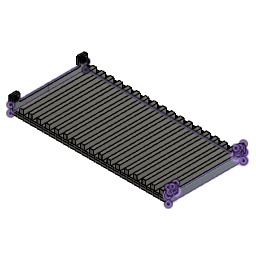
SSDTray v8 (Autodesk Fusion 360 archive; units mm, degrees)
design "SSDTray-Top"
Autodesk Fusion 360 part; units mm, degrees
sketch "PrimarySSD" plane through (0, 0, 0) normal (0, 1, 0) x (1, 0, 0)
  line L0 (0, 0) -> (7, 0)
  circle A0 centre (4, -14) radius 1.55
  circle A1 centre (4, -90.6) radius 1.55
  line L1 (0, 0) -> (-2.5, 0)
  line L2 (-2.5, 0) -> (-2.5, -100.45)
  line L3 (0, -100.45) -> (0, 0)
  line L4 (7, 0) -> (9.5, 0)
  line L5 (9.5, 0) -> (9.5, -100.45)
  line L6 (7, -100.45) -> (7, 0)
  line L7 (-2.5, -100.45) -> (9.5, -100.45)
  line L8 (-2.5, -100.45) -> (9.5, -100.45)
  line L9 (9.5, -100.45) -> (9.5, -102.95)
  line L10 (9.5, -102.95) -> (-2.5, -102.95)
  line L11 (-2.5, -102.95) -> (-2.5, -100.45)
  dimension "d1" = 7
  dimension "d3" = 3.1
  dimension "d5" = 14
  dimension "d6" = 3.1
  dimension "d8" = 90.6
  dimension "d10" = 100.45
  dimension "d12" = 100.45
  dimension "d17" = 2.5
  dimension "d18" = 2.5
  dimension "d19" = 12
  dimension "d20" = 3
  dimension "d21" = 3
  dimension "d44" = 9.85
  dimension "d92" = 12
  dimension "d93" = 2.5
  constraint horizontal L0
  constraint coincident L0.start L1.start
  constraint horizontal L1
  constraint vertical L2
  constraint vertical L3
  constraint horizontal L4
  constraint vertical L5
  constraint vertical L6
  constraint perpendicular L5 L7
  constraint horizontal L8
  constraint vertical L9
  constraint horizontal L10
  constraint vertical L11
  measures "d1" distance of L0.start L0.end
  measures "d3" diameter of A0
  measures "d5" distance of L0 A0.centre
  measures "d6" diameter of A1
  measures "d8" distance of L0 A1.centre
  measures "d10" distance of L0.start L3.start
  measures "d12" distance of L0.end L6.start
  measures "d17" distance of L2 L3
  measures "d18" distance of L5 L6
  measures "d19" distance of L2 L5
  measures "d20" distance of A1.centre L6
  measures "d21" distance of A0.centre L6
  measures "d44" distance of A1.centre L7
  measures "d92" distance of L2.end L5.end
  measures "d93" distance of L2.end L10.end
extrude "Extrude1" add sketch "PrimarySSD" along normal blind 10 contours L1 L2 L3 L7 L8 | L4 L5 L6 L7 L8 makes body 1 at (0, 3.3333, 66.9667) makes body 2 at (9.5, 3.3333, 33.4833)
extrude "Extrude6" add sketch "PrimarySSD" along normal blind 3 contours L0 L3 L6 L7 L8 bodies 1 2
ref_plane "WorkPlane2" through (3.5, 72.85, 50.225) normal (0, 1, 0) x (1, 0, 0)
sketch "TopSSD" plane through (0, 72.85, 0) normal (0, 1, 0) x (1, 0, 0)
  line L0 (-2.5, 0) -> (-2.5, -100.45)
  line L1 (0, -100.45) -> (0, 0)
  line L2 (7, -100.45) -> (7, 0)
  line L3 (9.5, 0) -> (9.5, -100.45)
  line L4 (-2.5, -100.45) -> (9.5, -100.45)
  line L5 (0, 0) -> (7, 0)
  line L6 (7, 0) -> (9.5, 0)
  line L7 (0, 0) -> (-2.5, 0)
  circle A0 centre (4, -14) radius 1.55
  circle A1 centre (4, -90.6) radius 1.55
  line L8 (9.5, -102.95) -> (-2.5, -102.95)
  line L9 (9.5, -100.45) -> (9.5, -102.95)
  line L10 (-2.5, -102.95) -> (-2.5, -100.45)
  point P0 (4, -14)
  point P1 (4, -90.6)
  point P2 (9.5, 0)
  point P3 (-2.5, 0)
  point P4 (9.5, -100.45)
extrude "Extrude12" add sketch "PrimarySSD" along normal blind 10 contours L7 L8 L9 L10 L11 bodies 1
pattern_linear "R-Pattern1" count 18 spacing 12 along (1, 0, 0) of bodies 1 makes body 3 at (15.6281, 0, 4.1514) makes body 4 at (27.6281, 0, 4.1514) makes body 5 at (39.6281, 0, 4.1514) makes body 6 at (51.6281, 0, 4.1514) makes body 7 at (63.6281, 0, 4.1514) makes body 8 at (75.6281, 0, 4.1514) makes body 9 at (87.6281, 0, 4.1514) makes body 10 at (99.6281, 0, 4.1514) makes body 11 at (111.6281, 0, 4.1514) makes body 12 at (123.6281, 0, 4.1514) makes body 13 at (135.6281, 0, 4.1514) makes body 14 at (147.6281, 0, 4.1514) makes body 15 at (159.6281, 0, 4.1514) makes body 16 at (171.6281, 0, 4.1514) makes body 17 at (183.6281, 0, 4.1514) makes body 18 at (195.6281, 0, 4.1514) makes body 19 at (207.6281, 0, 4.1514)
combine "Combine6" operation add target body 1 tool bodies 3 13 17 16 18 19 10 11 14 5 6 15 9 8 7 4 12
ref_plane "WorkPlane5" through (-2.5, 5, 51.475) normal (-1, 0, 0) x (0, 0, 1)
sketch "Left Mount" plane through (-2.5, 0, 0) normal (-1, 0, 0) x (0, 0, 1)
  line L0 (0, 0) -> (102.95, 0)
  line L1 (102.95, 0) -> (102.95, 10)
  line L2 (102.95, 10) -> (0, 10)
  line L3 (0, 10) -> (0, 0)
  line L4 (0, 10) -> (10, 10)
  line L5 (10, 10) -> (10, 20)
  line L6 (10, 20) -> (0, 20)
  line L7 (0, 20) -> (0, 10)
  line L8 (51.475, 0) -> (51.475, 10)
  line L9 (102.95, 20) -> (102.95, 10)
  line L10 (92.95, 20) -> (102.95, 20)
  line L11 (102.95, 10) -> (92.95, 10)
  line L12 (92.95, 10) -> (92.95, 20)
  circle A0 centre (5, 15) radius 1.625
  circle A1 centre (97.95, 15) radius 1.625
  line L13 (7.75, 16.5877) -> (5, 18.1754)
  line L14 (5, 18.1754) -> (2.25, 16.5877)
  line L15 (2.25, 16.5877) -> (2.25, 13.4123)
  line L16 (2.25, 13.4123) -> (5, 11.8246)
  line L17 (5, 11.8246) -> (7.75, 13.4123)
  line L18 (7.75, 13.4123) -> (7.75, 16.5877)
  line L19 (95.2, 16.5877) -> (97.95, 18.1754)
  line L20 (97.95, 18.1754) -> (100.7, 16.5877)
  line L21 (100.7, 16.5877) -> (100.7, 13.4123)
  line L22 (100.7, 13.4123) -> (97.95, 11.8246)
  line L23 (97.95, 11.8246) -> (95.2, 13.4123)
  line L24 (95.2, 13.4123) -> (95.2, 16.5877)
  point P0 (5, 15)
  dimension "d103" = 10
  dimension "d104" = 10
  dimension "d105" = 3.25
  dimension "d106" = 5
  dimension "d107" = 5
  dimension "d108" = 2.75
  constraint horizontal L4
  constraint vertical L5
  constraint horizontal L6
  constraint vertical L7
  constraint coincident L2.end L3.start
  constraint midpoint L0 L8.start
  constraint midpoint L2 L8.end
  constraint symmetric L2.end L8 L1.end
  constraint symmetric L4.end L8 L11.end
  constraint symmetric L5.end L8 L10.start
  constraint symmetric L6.end L8 L9.start
  constraint symmetric L8 A0 A1
  constraint coincident P0 A0.centre
  constraint vertical L15
  constraint symmetric L8 L13.start L19.start
  constraint symmetric L8 L13.end L19.end
  constraint symmetric L8 L14.end L20.end
  constraint symmetric L8 L15.end L21.end
  constraint symmetric L8 L16.end L22.end
  constraint symmetric L8 L17.end L23.end
  measures "d103" distance of L2.end L4.end
  measures "d104" distance of L2.end L6.end
  measures "d105" diameter of A0
  measures "d106" distance of L7 P0
  measures "d107" distance of L6 P0
  measures "d108" distance of P0 L18
extrude "Extrude15" add sketch "Left Mount" against normal blind 2.5 contours L2 L4 L5 L6 L7 bodies 1
extrude "Extrude16" add sketch "Left Mount" against normal blind 2.5 contours L2 L9 L10 L11 L12 bodies 1
extrude "Extrude17" add sketch "Left Mount" along normal blind 2.5 contours L2 L9 L10 L11 L12 | L19 L20 L21 L22 L23 L24 bodies 1
extrude "Extrude18" add sketch "Left Mount" along normal blind 2.5 contours L2 L4 L5 L6 L7 | L13 L14 L15 L16 L17 L18 bodies 1
ref_plane "WorkPlane6" through (213.5, 5, 51.475) normal (1, 0, 0) x (0, 0, -1)
sketch "Right Mount" plane through (213.5, 0, 0) normal (1, 0, 0) x (0, 0, -1)
  line L0 (-102.95, 0) -> (-102.95, 10)
  line L1 (0, 0) -> (-102.95, 0)
  line L2 (-102.95, 10) -> (0, 10)
  line L3 (0, 10) -> (0, 0)
  line L4 (0, 20) -> (0, 10)
  line L5 (-2.25, 16.5877) -> (-2.25, 13.4123)
  line L6 (-2.25, 13.4123) -> (-5, 11.8246)
  line L7 (-5, 11.8246) -> (-7.75, 13.4123)
  line L8 (-7.75, 13.4123) -> (-7.75, 16.5877)
  line L9 (-7.75, 16.5877) -> (-5, 18.1754)
  line L10 (-5, 18.1754) -> (-2.25, 16.5877)
  circle A0 centre (-5, 15) radius 1.625
  line L11 (-10, 20) -> (0, 20)
  line L12 (-10, 10) -> (-10, 20)
  line L13 (-92.95, 10) -> (-92.95, 20)
  line L14 (-92.95, 20) -> (-102.95, 20)
  line L15 (-102.95, 20) -> (-102.95, 10)
  line L16 (-100.7, 16.5877) -> (-100.7, 13.4123)
  line L17 (-100.7, 13.4123) -> (-97.95, 11.8246)
  line L18 (-97.95, 11.8246) -> (-95.2, 13.4123)
  line L19 (-95.2, 13.4123) -> (-95.2, 16.5877)
  line L20 (-95.2, 16.5877) -> (-97.95, 18.1754)
  line L21 (-97.95, 18.1754) -> (-100.7, 16.5877)
  circle A1 centre (-97.95, 15) radius 1.625
  point P0 (-5, 15)
  point P1 (-97.95, 15)
extrude "Extrude19" add sketch "Right Mount" against normal blind 2.5 contours L2 L13 L14 L15 bodies 1
extrude "Extrude20" add sketch "Right Mount" along normal blind 2.5 contours L2 L13 L14 L15 | L16 L17 L18 L19 L20 L21 bodies 1
extrude "Extrude21" add sketch "Right Mount" against normal blind 2.5 contours L2 L4 L11 L12 bodies 1
extrude "Extrude22" add sketch "Right Mount" along normal blind 2.5 contours L2 L4 L11 L12 | L5 L6 L7 L8 L9 L10 bodies 1
sketch "Sketch13" plane through (0, 10, 0) normal (0, 1, 0) x (-1, 0, 0)
  line L0 (-211, 102.95) -> (-211, 100.45)
  line L1 (-211, 100.45) -> (-204, 100.45)
  line L2 (-204, 100.45) -> (-204, 0)
  line L3 (-204, 0) -> (-199, 0)
  line L4 (-199, 0) -> (-199, 100.45)
  line L5 (-199, 100.45) -> (-192, 100.45)
  line L6 (-192, 100.45) -> (-192, 0)
  line L7 (-192, 0) -> (-187, 0)
  line L8 (-187, 0) -> (-187, 100.45)
  line L9 (-187, 100.45) -> (-180, 100.45)
  line L10 (-180, 100.45) -> (-180, 0)
  line L11 (-180, 0) -> (-175, 0)
  line L12 (-175, 0) -> (-175, 100.45)
  line L13 (-175, 100.45) -> (-168, 100.45)
  line L14 (-168, 100.45) -> (-168, 0)
  line L15 (-168, 0) -> (-163, 0)
  line L16 (-163, 0) -> (-163, 100.45)
  line L17 (-163, 100.45) -> (-156, 100.45)
  line L18 (-156, 100.45) -> (-156, 0)
  line L19 (-156, 0) -> (-151, 0)
  line L20 (-151, 0) -> (-151, 100.45)
  line L21 (-151, 100.45) -> (-144, 100.45)
  line L22 (-144, 100.45) -> (-144, 0)
  line L23 (-144, 0) -> (-139, 0)
  line L24 (-139, 0) -> (-139, 100.45)
  line L25 (-139, 100.45) -> (-132, 100.45)
  line L26 (-132, 100.45) -> (-132, 0)
  line L27 (-132, 0) -> (-127, 0)
  line L28 (-127, 0) -> (-127, 100.45)
  line L29 (-127, 100.45) -> (-120, 100.45)
  line L30 (-120, 100.45) -> (-120, 0)
  line L31 (-120, 0) -> (-115, 0)
  line L32 (-115, 0) -> (-115, 100.45)
  line L33 (-115, 100.45) -> (-108, 100.45)
  line L34 (-108, 100.45) -> (-108, 0)
  line L35 (-108, 0) -> (-103, 0)
  line L36 (-103, 0) -> (-103, 100.45)
  line L37 (-103, 100.45) -> (-96, 100.45)
  line L38 (-96, 100.45) -> (-96, 0)
  line L39 (-96, 0) -> (-91, 0)
  line L40 (-91, 0) -> (-91, 100.45)
  line L41 (-91, 100.45) -> (-84, 100.45)
  line L42 (-84, 100.45) -> (-84, 0)
  line L43 (-84, 0) -> (-79, 0)
  line L44 (-79, 0) -> (-79, 100.45)
  line L45 (-79, 100.45) -> (-72, 100.45)
  line L46 (-72, 100.45) -> (-72, 0)
  line L47 (-72, 0) -> (-67, 0)
  line L48 (-67, 0) -> (-67, 100.45)
  line L49 (-67, 100.45) -> (-60, 100.45)
  line L50 (-60, 100.45) -> (-60, 0)
  line L51 (-60, 0) -> (-55, 0)
  line L52 (-55, 0) -> (-55, 100.45)
  line L53 (-55, 100.45) -> (-48, 100.45)
  line L54 (-48, 100.45) -> (-48, 0)
  line L55 (-48, 0) -> (-43, 0)
  line L56 (-43, 0) -> (-43, 100.45)
  line L57 (-43, 100.45) -> (-36, 100.45)
  line L58 (-36, 100.45) -> (-36, 0)
  line L59 (-36, 0) -> (-31, 0)
  line L60 (-31, 0) -> (-31, 100.45)
  line L61 (-31, 100.45) -> (-24, 100.45)
  line L62 (-24, 100.45) -> (-24, 0)
  line L63 (-24, 0) -> (-19, 0)
  line L64 (-19, 0) -> (-19, 100.45)
  line L65 (-19, 100.45) -> (-12, 100.45)
  line L66 (-12, 100.45) -> (-12, 0)
  line L67 (-12, 0) -> (-7, 0)
  line L68 (-7, 0) -> (-7, 100.45)
  line L69 (-7, 100.45) -> (0, 100.45)
  line L70 (0, 100.45) -> (0, 102.95)
  line L71 (0, 102.95) -> (-211, 102.95)
  line L72 (2.5, 102.95) -> (-15.75, 102.95)
  line L73 (-7, 100.45) -> (0, 100.45)
  line L74 (-19, 100.45) -> (-12, 100.45)
  line L75 (-211, 102.95) -> (0, 102.95)
  line L76 (-31, 100.45) -> (-24, 100.45)
  line L77 (-43, 100.45) -> (-36, 100.45)
  line L78 (0, 102.95) -> (-211, 102.95)
  line L79 (-211, 102.95) -> (-211, 100.45)
  line L80 (-211, 100.45) -> (0, 100.45)
  line L81 (0, 100.45) -> (0, 102.95)
  line L82 (-211, 102.95) -> (-211, 100.45)
  line L83 (-211, 100.45) -> (-204, 100.45)
  line L84 (-204, 100.45) -> (-204, 0)
  line L85 (-204, 0) -> (-199, 0)
  line L86 (-199, 0) -> (-199, 100.45)
  line L87 (-199, 100.45) -> (-192, 100.45)
  line L88 (-192, 100.45) -> (-192, 0)
  line L89 (-192, 0) -> (-187, 0)
  line L90 (-187, 0) -> (-187, 100.45)
  line L91 (-187, 100.45) -> (-180, 100.45)
  line L92 (-180, 100.45) -> (-180, 0)
  line L93 (-180, 0) -> (-175, 0)
  line L94 (-175, 0) -> (-175, 100.45)
  line L95 (-175, 100.45) -> (-168, 100.45)
  line L96 (-168, 100.45) -> (-168, 0)
  line L97 (-168, 0) -> (-163, 0)
  line L98 (-163, 0) -> (-163, 100.45)
  line L99 (-163, 100.45) -> (-156, 100.45)
  line L100 (-156, 100.45) -> (-156, 0)
  line L101 (-156, 0) -> (-151, 0)
  line L102 (-151, 0) -> (-151, 100.45)
  line L103 (-151, 100.45) -> (-144, 100.45)
  line L104 (-144, 100.45) -> (-144, 0)
  line L105 (-144, 0) -> (-139, 0)
  line L106 (-139, 0) -> (-139, 100.45)
  line L107 (-139, 100.45) -> (-132, 100.45)
  line L108 (-132, 100.45) -> (-132, 0)
  line L109 (-132, 0) -> (-127, 0)
  line L110 (-127, 0) -> (-127, 100.45)
  line L111 (-127, 100.45) -> (-120, 100.45)
  line L112 (-120, 100.45) -> (-120, 0)
  line L113 (-120, 0) -> (-115, 0)
  line L114 (-115, 0) -> (-115, 100.45)
  line L115 (-115, 100.45) -> (-108, 100.45)
  line L116 (-108, 100.45) -> (-108, 0)
  line L117 (-108, 0) -> (-103, 0)
  line L118 (-103, 0) -> (-103, 100.45)
  line L119 (-103, 100.45) -> (-96, 100.45)
  line L120 (-96, 100.45) -> (-96, 0)
  line L121 (-96, 0) -> (-91, 0)
  line L122 (-91, 0) -> (-91, 100.45)
  line L123 (-91, 100.45) -> (-84, 100.45)
  line L124 (-84, 100.45) -> (-84, 0)
  line L125 (-84, 0) -> (-79, 0)
  line L126 (-79, 0) -> (-79, 100.45)
  line L127 (-79, 100.45) -> (-72, 100.45)
  line L128 (-72, 100.45) -> (-72, 0)
  line L129 (-72, 0) -> (-67, 0)
  line L130 (-67, 0) -> (-67, 100.45)
  line L131 (-67, 100.45) -> (-60, 100.45)
  line L132 (-60, 100.45) -> (-60, 0)
  line L133 (-60, 0) -> (-55, 0)
  line L134 (-55, 0) -> (-55, 100.45)
  line L135 (-55, 100.45) -> (-48, 100.45)
  line L136 (-48, 100.45) -> (-48, 0)
  line L137 (-48, 0) -> (-43, 0)
  line L138 (-43, 0) -> (-43, 100.45)
  line L139 (-43, 100.45) -> (-36, 100.45)
  line L140 (-36, 100.45) -> (-36, 0)
  line L141 (-36, 0) -> (-31, 0)
  line L142 (-31, 0) -> (-31, 100.45)
  line L143 (-31, 100.45) -> (-24, 100.45)
  line L144 (-24, 100.45) -> (-24, 0)
  line L145 (-24, 0) -> (-19, 0)
  line L146 (-19, 0) -> (-19, 100.45)
  line L147 (-19, 100.45) -> (-12, 100.45)
  line L148 (-12, 100.45) -> (-12, 0)
  line L149 (-12, 0) -> (-7, 0)
  line L150 (-7, 0) -> (-7, 100.45)
  line L151 (-7, 100.45) -> (0, 100.45)
  line L152 (0, 100.45) -> (0, 102.95)
  line L153 (0, 102.95) -> (-211, 102.95)
  dimension "d187" = 211
  dimension "d188" = 2.5
  constraint horizontal L78
  constraint vertical L79
  constraint horizontal L80
  constraint vertical L81
  constraint coincident L70.end L71.start
  measures "d187" distance of L70.end L0.start
  measures "d188" distance of L70.end L69.end
extrude "Extrude35" cut sketch "Sketch13" against normal blind 6.5 contours L0 L1 L5 L9 L13 L17 L21 L25 L29 L33 L37 L41 L45 L49 L53 L57 L61 L65 L69 L70 L71 L72 L73 L74 L75 L76 L77 L78 L79 L80 L81 L82 L83 L87 L91 L95 L99 L103 L107 L111 L115 L119 L123 L127 L131 L135 L139 L143 L147 L151 L152 L153 bodies 1
sketch "Sketch14" plane through (0, 0, 0) normal (0, 1, 0) x (1, 0, 0)
  line L0 (-2.5, 0) -> (213.5, 0)
  line L1 (-2.5, 0) -> (213.5, 0)
  line L2 (213.5, 0) -> (213.5, 1.6)
  line L3 (213.5, 1.6) -> (-2.5, 1.6)
  line L4 (-2.5, 1.6) -> (-2.5, 0)
  line L5 (-2.5, 0) -> (213.5, 0)
  line L6 (213.5, 0) -> (213.5, 2.5)
  line L7 (213.5, 2.5) -> (-2.5, 2.5)
  line L8 (-2.5, 2.5) -> (-2.5, 0)
  dimension "d191" = 216
  dimension "d192" = 1.6
  dimension "d193" = 2.5
  constraint horizontal L1
  constraint vertical L2
  constraint horizontal L3
  constraint vertical L4
  constraint coincident L0.start L1.start
  constraint horizontal L5
  constraint vertical L6
  constraint horizontal L7
  constraint vertical L8
  measures "d191" distance of L0.start L0.end
  measures "d192" distance of L0.start L3.end
  measures "d193" distance of L0.start L7.end
extrude "Extrude36" add sketch "Sketch14" along normal blind 3 bodies 1
extrude "Extrude37" add sketch "Sketch14" along normal blind 5 contours L3 L6 L7 L8 bodies 1
named bodies: "BottomTray"

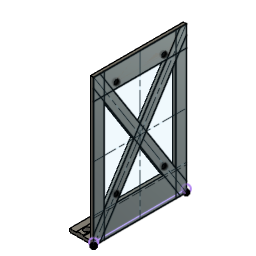
design "2U Ears"
Autodesk Fusion 360 part; units mm, degrees
sketch "Sketch1" plane through (0, 0, 0) normal (0, 1, 0) x (1, 0, 0)
  line L0 (0, 0) -> (-20, 0)
  line L1 (-20, 0) -> (-20, -44.45)
  line L2 (-20, -44.45) -> (0, -44.45)
  line L3 (0, -44.45) -> (0, 0)
  line L4 (-10, 0) -> (-10, -44.45)
  circle A0 centre (-10, -6.35) radius 3.05
  circle A1 centre (-10, -22.225) radius 3.05
  circle A2 centre (-10, -38.1) radius 3.05
  line L5 (-6.9, -44.45) -> (-13.1, -44.45)
  line L6 (-13.1, -44.45) -> (-13.1, 0)
  line L7 (-13.1, 0) -> (-6.9, 0)
  line L8 (-6.9, 0) -> (-6.9, -44.45)
  line L9 (-6.9, -44.45) -> (-13.1, 0) construction
  line L10 (-13.1, -44.45) -> (-6.9, 0) construction
  line L11 (0, 0) -> (3, 0)
  line L12 (3, 0) -> (3, -44.45)
  line L13 (3, -44.45) -> (0, -44.45)
  line L14 (0, -44.45) -> (0, 0)
  point P0 (-10, -22.225)
  dimension "d1" = 20
  dimension "d2" = 44.45
  dimension "d3" = 6.1
  dimension "d4" = 6.35
  dimension "d5" = 6.1
  dimension "d6" = 15.875
  dimension "d7" = 6.1
  dimension "d8" = 15.875
  dimension "d9" = 6.35
  dimension "d10" = 6.2
  dimension "d11" = 44.45
  dimension "d12" = 3
  dimension "d13" = 44.45
  constraint horizontal L0
  constraint vertical L1
  constraint horizontal L2
  constraint vertical L3
  constraint coincident L0.start L3.end
  constraint midpoint L0 L4.start
  constraint midpoint L2 L4.end
  constraint coincident L4 A0.centre
  constraint coincident L4 P0
  constraint coincident L4 A2.centre
  constraint horizontal L5
  constraint perpendicular L5 L6
  constraint parallel L5 L7
  constraint parallel L6 L8
  constraint coincident L9 P0
  constraint coincident L10 P0
  constraint coincident P0 A1.centre
  constraint horizontal L11
  constraint vertical L12
  constraint horizontal L13
  constraint vertical L14
  measures "d1" distance of L0.start L0.end
  measures "d2" distance of L0 L2
  measures "d3" diameter of A0
  measures "d4" distance of L4.start A0.centre
  measures "d5" diameter of A1
  measures "d6" distance of A0.centre P0
  measures "d7" diameter of A2
  measures "d8" distance of P0 A2.centre
  measures "d9" distance of L2 A2.centre
  measures "d10" distance of L6.end L7.end
  measures "d11" distance of L5.end L6.end
  measures "d12" distance of L0.start L11.end
  measures "d13" distance of L0.start L2.end
extrude "Extrude1" add sketch "Sketch1" along normal blind 3 contours L0 L2 L3 L8 L14 | L3 L11 L12 L13 L14 | L0 L2 L4 A0 A1 A2 L5 L7 L8 | L0 L2 L4 A0 A1 A2 L5 L6 L7 | L0 L1 L2 L6 makes body 1
extrude "Extrude2" add sketch "Sketch1" along normal blind 25 contours L3 L11 L12 L13 L14 bodies 1
extrude "Extrude3" add sketch "Sketch1" along normal blind 4 separate body contours L0 L2 L4 A0 A1 A2 L5 L7 L8 | L0 L2 L4 A0 A1 A2 L5 L6 L7 makes body 2
combine "Combine1" operation add target body 1 tool bodies 2
pattern_linear "R-Pattern1" count 1 spacing 0 along (1, 0, 0) count 2 spacing 44.45 along (0, 0, 1) of bodies 1 makes body 3
combine "Combine2" operation add target body 1 tool bodies 3
sketch "Sketch2" plane through (3, 0, 0) normal (1, 0, 0) x (0, 0, -1)
  line L0 (-88.9, 0) -> (0, 0)
  line L1 (0, 0) -> (0, 25)
  line L2 (0, 25) -> (-88.9, 25)
  line L3 (-88.9, 25) -> (-88.9, 0)
  line L4 (-88.9, 0) -> (0, 0)
  line L5 (0, 0) -> (0, 140)
  line L6 (0, 140) -> (-88.9, 140)
  line L7 (-88.9, 140) -> (-88.9, 0)
  line L8 (-44.45, 140) -> (-44.45, 0)
  line L9 (-88.9, 70) -> (0, 70)
  line L10 (0, 140) -> (-88.9, 0)
  line L11 (-88.9, 140) -> (0, 0)
  line L12 (-88.9, 9.3274) -> (-5.9229, 140)
  line L13 (-82.9771, 0) -> (0, 130.6726)
  line L14 (-82.9771, 140) -> (0, 9.3274)
  line L15 (-5.9229, 0) -> (-88.9, 130.6726)
  line L16 (-78.9, 140) -> (-78.9, 0)
  line L17 (-10, 140) -> (-10, 0)
  line L18 (-88.9, 3) -> (0, 3)
  line L19 (-88.9, 23) -> (0, 23) construction
  line L20 (-88.9, 25) -> (0, 25) construction
  circle A0 centre (-67.375, 32.5) radius 1.625
  circle A1 centre (-21.525, 32.5) radius 1.625
  circle A2 centre (-21.525, 125.425) radius 1.625
  circle A3 centre (-67.375, 125.425) radius 1.625
  line L21 (-88.9, 120) -> (0, 120)
  dimension "d24" = 88.9
  dimension "d25" = 140
  dimension "d26" = 10
  dimension "d27" = 10
  dimension "d28" = 10
  dimension "d29" = 10
  dimension "d30" = 10
  dimension "d31" = 10
  dimension "d32" = 20
  dimension "d33" = 25
  dimension "d34" = 3.25
  dimension "d35" = 7.5
  dimension "d36" = 3.25
  dimension "d37" = 7.5
  dimension "d40" = 45.85
  dimension "d41" = 45.85
  dimension "d42" = 3.25
  dimension "d43" = 92.925
  dimension "d44" = 45.85
  dimension "d45" = 3.25
  dimension "d46" = 92.925
  dimension "d47" = 45.85
  dimension "d48" = 20
  constraint horizontal L4
  constraint vertical L5
  constraint horizontal L6
  constraint vertical L7
  constraint coincident L0.start L3.end
  constraint midpoint L6 L8.start
  constraint midpoint L4 L8.end
  constraint midpoint L7 L9.start
  constraint midpoint L5 L9.end
  constraint coincident L0.end L1.start
  constraint coincident L7 L12.start
  constraint coincident L6 L12.end
  constraint parallel L10 L12
  constraint coincident L4 L13.start
  constraint coincident L5 L13.end
  constraint parallel L10 L13
  constraint coincident L6 L14.start
  constraint coincident L5 L14.end
  constraint coincident L4 L15.start
  constraint coincident L7 L15.end
  constraint parallel L11 L15
  constraint parallel L11 L14
  constraint coincident L6 L16.start
  constraint coincident L4 L16.end
  constraint perpendicular L4 L16
  constraint coincident L6 L17.start
  constraint coincident L4 L17.end
  constraint perpendicular L4 L17
  constraint coincident L7 L19.start
  constraint coincident L5 L19.end
  constraint perpendicular L5 L19
  constraint coincident L7 L2.end
  constraint coincident L5 L1.end
  constraint perpendicular L5 L20
  constraint coincident L7 L21.start
  constraint coincident L5 L21.end
  constraint perpendicular L5 L21
  measures "d24" distance of L0.start L0.end
  measures "d25" distance of L0.start L6.end
  measures "d30" distance of L7 L16
  measures "d31" distance of L5 L17
  measures "d32" distance of L18 L19
  measures "d33" distance of L4 L20
  measures "d34" diameter of A0
  measures "d35" distance of L20 A0.centre
  measures "d36" diameter of A1
  measures "d37" distance of L20 A1.centre
  measures "d42" diameter of A2
  measures "d43" vertical distance of A1.centre A2.centre
  measures "d45" diameter of A3
  measures "d46" vertical distance of A0.centre A3.centre
  measures "d48" distance of L6 L21
extrude "Extrude4" add sketch "Sketch2" against normal blind 3 contours L2 L7 L9 L12 L16 | L2 L12 L16 | L2 L10 L13 L15 A0 | L2 L10 L12 L15 L16 A0 | L7 L9 L15 L16 L21 | L8 L10 L15 | L8 L11 L13 | L2 L11 L13 L15 A1 | L7 L15 L21 | L9 L11 L12 | L11 L12 L15 L16 L21 | L9 L10 L15 | L8 L11 L12 | L9 L10 L14 | L8 L10 L14 | L9 L11 L13 | L2 L11 L13 L14 L17 A1 | L7 L11 L15 L16 L21 | L15 L16 L21 | L11 L12 L14 L21 | L10 L12 L14 L21 | L10 L13 L14 L17 L21 | L6 L11 L14 L16 | L11 L14 L16 L21 | L2 L14 L17 | L6 L8 L14 L16 L21 | L6 L8 L12 L17 L21 | L10 L12 L17 L21 | L5 L9 L13 L17 L21 | L2 L5 L9 L14 L17 | L13 L17 L21 | L6 L14 L16 | L6 L12 L17 | L6 L10 L12 L17 | L5 L10 L13 L17 L21 | L5 L13 L21 bodies 1
extrude "Extrude5" add sketch "Sketch2" against normal blind 3 contours L10 L17 L21 bodies 1
extrude "Extrude6" add sketch "Sketch2" against normal blind 3 contours L11 L16 L21 bodies 1

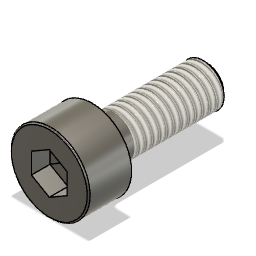
design "Socket Head Cap Screw JIS B 1176 - M3 x 0.5 x 8 Steel 4.6 Plain"
description: Socket Head Cap Screw JIS B 1176 - M3 x 0.5 x 8
Autodesk Fusion 360 part; units mm, degrees
sketch "Sketch1" plane through (0, 0, 0) normal (0, 1, 0) x (1, 0, 0)
  line L0 (-1.5, 0) -> (-1.5, 8)
  line L1 (-1.5, 8) -> (0, 8)
  line L2 (0, 8) -> (0, -3)
  line L3 (-1.5, 0) -> (-2.75, 0)
  line L4 (-2.75, 0) -> (-2.75, -3)
  line L5 (-2.75, -3) -> (0, -3)
  dimension "d9" = 3
  dimension "d66" = 5.5
  dimension "d68" = 8
  dimension "d79" = 3
  constraint perpendicular L0 L1
  constraint collinear origin L1.end L2.end
  constraint perpendicular L0 L3
  constraint coincident origin L3
  constraint vertical L0
  constraint vertical L2
  constraint parallel L2 L4
  constraint coincident L2 L5.end
  constraint perpendicular L2 L5
  measures "d68" distance of origin L1.end
  measures "d79" distance of L3.end L4.end
revolve "Revolve1" add sketch "Sketch1" angle 360 about axis through (0, 0, -8) along (0, 0, 1)
ref_plane "WorkPlane1" through (0, 0, 3) normal (0, 0, 1) x (1, 0, 0)
sketch "Sketch6" plane through (0, 0, 3) normal (0, 0, 1) x (1, 0, 0)
  line L0 (-1.25, 0) -> (1.25, 0) construction
  line L1 (0, 0) -> (-1.25, 0.7217)
  line L2 (-1.25, -0.7217) -> (-1.25, 0.7217)
  line L3 (-1.25, -0.7217) -> (0, 0)
  dimension "d72" = 2.5
  dimension "d97" = 150
  constraint horizontal L0
  constraint midpoint L1.start L0
  constraint coincident L1.start L3.end
  constraint perpendicular L0 L2
  constraint midpoint L0.start L2
  constraint coincident L1.end L2.end
  measures "d72" distance of L0.start L0.end
  measures "d97" angle of L0 L1
extrude "Extrude1" cut sketch "Sketch6" against normal blind 1.3
pattern_circular "C-Pattern1" count 6 over 360 about axis through (0, 0, 1.75) along (0, 0, 1) of "Extrude1"
extrude "Extrude2" cut 1 faces at (0, 0.4811, 1.7) along direction (0, 0, -1) blind 1.3 draft -85
thread "Thread2" "ISO Metric profile 3.0 M3x0.5 6g" major diameter 2.927 minor diameter 2.3555 pitch 0.5 angle 60 resizes the face on face at (-1.4981, 0.0748, -5.3333) from (0, 0, -1.5) to (0, 0, -8)
sketch "Sketch7" plane through (0, 0, 0) normal (0, 1, 0) x (1, 0, 0)
  line L0 (-1.53, 8) -> (-1.53, 7.6933)
  line L1 (-1.53, 7.6933) -> (-1.1933, 8)
  line L2 (0, 8) -> (0, -3)
  line L3 (-1.53, 8) -> (0, 8)
  dimension "d94" = 1.53
  dimension "d95" = 0.3067
  dimension "d96" = 1.1933
  constraint coincident L2.start L3.end
  constraint perpendicular L0 L3
  constraint coincident L1.end L3
  constraint perpendicular L2 L3
  measures "d94" distance of origin L0
  measures "d95" vertical distance of L0.end L1.end
  measures "d96" horizontal distance of origin L1.end
revolve "Revolve3" cut sketch "Sketch7" angle 360 about axis through (0, 0, 1.75) along (0, 0, 1)
fillet "Fillet5" radius 0.1 1 edges at (-2.5639, 0.9944, 3)
fillet "Fillet7" radius 0.3 1 edges at (1.3645, -0.5292, 0)
equation "d9 = adsk_nomdia"
equation "adsk_nomlen = 8.00 mm"
equation "adsk_headh = 3.00 mm"
equation "adsk_headdia = 5.50 mm"
equation "adsk_nomdia = 3.00 mm"
equation "adsk_philwidth = 2.50 mm"
equation "d31 = -adsk_phildepth"
equation "adsk_phildepth = 1.30 mm"
equation "d66 = adsk_headdia"
equation "d68 = adsk_nomlen"
equation "d71 = adsk_headh"
equation "d72 = adsk_philwidth"
equation "d76 = -adsk_phildepth"
equation "d79 = adsk_headh"
equation "adsk_thrlen = 6.50 mm"
equation "d84 = adsk_thrlen"
equation "adsk_startlen = 0.306725 mm"
equation "adsk_endpointdia = 2.38655 mm"
equation "d94 = adsk_nomdia * 0.51"
equation "d95 = adsk_startlen"
equation "d96 = adsk_endpointdia / 2"
equation "adsk_headtoprad = 0.10 mm"
equation "d102 = adsk_headtoprad"
equation "adsk_midfillet = 0.30 mm"
equation "d107 = adsk_midfillet"

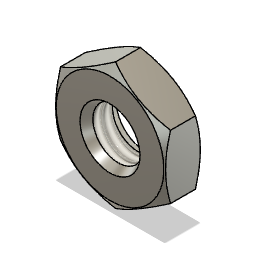
design "Hexagon Thin Nut DIN 439-2 - M3 x 0.5 Steel 6 Plain"
description: Hexagon Thin Nut DIN 439-2 - M3 x 0.5
Autodesk Fusion 360 part; units mm, degrees
sketch "Sketch1" plane through (0, 0, 0) normal (0, 1, 0) x (1, 0, 0)
  line L0 (0, 0) -> (0, -1.8)
  line L1 (-1.5, 0) -> (-2.695, 0)
  line L2 (-2.695, 0) -> (-3.1763, -0.2778)
  line L3 (-3.1763, -0.2778) -> (-3.1763, -1.5222)
  line L4 (-3.1763, -1.5222) -> (-2.695, -1.8)
  line L5 (-2.695, -1.8) -> (-1.5, -1.8)
  line L6 (-1.5, -1.8) -> (-1.5, 0)
  dimension "d121" = 3
  dimension "d122" = 30
  dimension "d123" = 30
  dimension "d126" = 1.8
  dimension "d128" = 6.3525
  dimension "d172" = 5.39
  constraint vertical L0
  constraint coincident L0 L0.end
  constraint coincident origin L0
  constraint horizontal L1
  constraint perpendicular L1 L3
  constraint perpendicular L3 L5
  constraint perpendicular L5 L6
  constraint coincident L0.start L1
  constraint coincident L0.start origin
  constraint coincident L0.end L5
  constraint equal L1 L5
  measures "d122" angle of L1 L2
  measures "d123" angle of L4 L5
  measures "d126" distance of L1.start L5.end
revolve "Revolve1" add sketch "Sketch1" angle 360 about axis through (0, 0, 0) along (0, 0, 1)
sketch "Sketch8" plane through (0, 0, 1.8) normal (0, 0, 1) x (1, 0, 0)
  line L0 (0, 0) -> (-5.5, 0) construction
  line L1 (-2.75, -1.5894) -> (-2.75, 1.5894)
  circle A0 centre (0, 0) radius 1.5
  circle A1 centre (0, 0) radius 3.1763
  dimension "d114" = 2.75
  constraint horizontal L0
  constraint perpendicular L0 L1
  constraint midpoint L0 L1
  constraint coincident L0.start A0.centre
  constraint coincident L1.end A1
  measures "d114" distance of L0.start L1
extrude "Extrude5" cut sketch "Sketch8" against normal blind 1.8 contours L1 A1 picked at (-2.8188, 0.3871)
pattern_circular "C-Pattern2" count 6 over 360 about axis through (0, 0, 1.75) along (0, 0, 1) of "Extrude5"
thread "Thread3" "ISO Metric profile 3.0 M3x0.5 6H" major diameter 3.086 minor diameter 2.529 pitch 0.5 angle 60 resizes the face on face at (-1.4981, 0.0748, 1.2)
sketch "Sketch12" plane through (0, 0, 0) normal (0, 1, 0) x (1, 0, 0)
  line L0 (1.2645, -1.8) -> (-1.2645, -1.8)
  line L1 (2.695, -1.8) -> (-2.695, -1.8)
  line L2 (2.695, 0) -> (-2.695, 0)
  line L3 (1.2645, 0) -> (-1.2645, 0)
  line L4 (-1.5, 0) -> (0, 0)
  line L5 (-0.9804, -0.9) -> (-1.5, 0)
  line L6 (-1.5, -1.8) -> (0, -1.8)
  line L7 (-0.9804, -0.9) -> (-1.5, -1.8)
  line L8 (0, 0) -> (0, -1.8)
  dimension "d165" = 60
  dimension "d169" = 60
  dimension "d170" = 1.5
  constraint horizontal L4
  constraint collinear L1 L6
  constraint coincident L5.start L7.start
  constraint vertical L4.start L6.start
  constraint coincident L1 L6.end
  constraint coincident L6.end L8.end
  constraint coincident L4.end L8.start
  measures "d165" angle of L2 L5
  measures "d169" angle of L6 L7
  measures "d170" distance of L4.start L4.end
revolve "Revolve3" cut sketch "Sketch12" angle 360 about axis through (0, 0, 1.75) along (0, 0, 1)
equation "adsk_nheig = 1.80 mm"
equation "adsk_maxdia = 6.3525 mm"
equation "adsk_nomdia = 3.00 mm"
equation "d89 = -adsk_nheig"
equation "adsk_waflat = 5.50 mm"
equation "d114 = adsk_waflat / 2"
equation "adsk_chamang1 = 30.00 deg"
equation "adsk_chamang2 = 30.00 deg"
equation "d121 = adsk_nomdia"
equation "d122 = adsk_chamang1"
equation "d123 = adsk_chamang2"
equation "d126 = adsk_nheig"
equation "d128 = adsk_maxdia"
equation "d163 = adsk_nheig"
equation "d170 = adsk_nomdia * 0.5"
equation "adsk_beardia = adsk_waflat * 0.98"
equation "d172 = adsk_beardia"

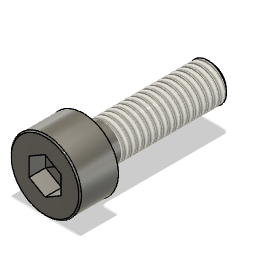
design "Socket Head Cap Screw JIS B 1176 - M3 x 0.5 x 10 Steel 4.6 Plain"
description: Socket Head Cap Screw JIS B 1176 - M3 x 0.5 x 10
Autodesk Fusion 360 part; units mm, degrees
sketch "Sketch1" plane through (0, 0, 0) normal (0, 1, 0) x (1, 0, 0)
  line L0 (-1.5, 0) -> (-1.5, 10)
  line L1 (-1.5, 10) -> (0, 10)
  line L2 (0, 10) -> (0, -3)
  line L3 (-1.5, 0) -> (-2.75, 0)
  line L4 (-2.75, 0) -> (-2.75, -3)
  line L5 (-2.75, -3) -> (0, -3)
  dimension "d9" = 3
  dimension "d66" = 5.5
  dimension "d68" = 10
  dimension "d79" = 3
  constraint perpendicular L0 L1
  constraint collinear origin L1.end L2.end
  constraint perpendicular L0 L3
  constraint coincident origin L3
  constraint vertical L0
  constraint vertical L2
  constraint parallel L2 L4
  constraint coincident L2 L5.end
  constraint perpendicular L2 L5
  measures "d68" distance of origin L1.end
  measures "d79" distance of L3.end L4.end
revolve "Revolve1" add sketch "Sketch1" angle 360 about axis through (0, 0, -10) along (0, 0, 1)
ref_plane "WorkPlane1" through (0, 0, 3) normal (0, 0, 1) x (1, 0, 0)
sketch "Sketch6" plane through (0, 0, 3) normal (0, 0, 1) x (1, 0, 0)
  line L0 (-1.25, 0) -> (1.25, 0) construction
  line L1 (0, 0) -> (-1.25, 0.7217)
  line L2 (-1.25, -0.7217) -> (-1.25, 0.7217)
  line L3 (-1.25, -0.7217) -> (0, 0)
  dimension "d72" = 2.5
  dimension "d97" = 150
  constraint horizontal L0
  constraint midpoint L1.start L0
  constraint coincident L1.start L3.end
  constraint perpendicular L0 L2
  constraint midpoint L0.start L2
  constraint coincident L1.end L2.end
  measures "d72" distance of L0.start L0.end
  measures "d97" angle of L0 L1
extrude "Extrude1" cut sketch "Sketch6" against normal blind 1.3
pattern_circular "C-Pattern1" count 6 over 360 about axis through (0, 0, 1.75) along (0, 0, 1) of "Extrude1"
extrude "Extrude2" cut 1 faces at (0, 0.4811, 1.7) along direction (0, 0, -1) blind 1.3 draft -85
thread "Thread2" "ISO Metric profile 3.0 M3x0.5 6g" major diameter 2.927 minor diameter 2.3555 pitch 0.5 angle 60 resizes the face on face at (-1.4925, 0.1494, -6.6667) from (0, 0, -1.5) to (0, 0, -10)
sketch "Sketch7" plane through (0, 0, 0) normal (0, 1, 0) x (1, 0, 0)
  line L0 (-1.53, 10) -> (-1.53, 9.6933)
  line L1 (-1.53, 9.6933) -> (-1.1933, 10)
  line L2 (0, 10) -> (0, -3)
  line L3 (-1.53, 10) -> (0, 10)
  dimension "d94" = 1.53
  dimension "d95" = 0.3067
  dimension "d96" = 1.1933
  constraint coincident L2.start L3.end
  constraint perpendicular L0 L3
  constraint coincident L1.end L3
  constraint perpendicular L2 L3
  measures "d94" distance of origin L0
  measures "d95" vertical distance of L0.end L1.end
  measures "d96" horizontal distance of origin L1.end
revolve "Revolve3" cut sketch "Sketch7" angle 360 about axis through (0, 0, 1.75) along (0, 0, 1)
fillet "Fillet5" radius 0.1 1 edges at (-2.5639, 0.9944, 3)
fillet "Fillet7" radius 0.3 1 edges at (1.3645, -0.5292, 0)
equation "d9 = adsk_nomdia"
equation "adsk_nomlen = 10.00 mm"
equation "adsk_headh = 3.00 mm"
equation "adsk_headdia = 5.50 mm"
equation "adsk_nomdia = 3.00 mm"
equation "adsk_philwidth = 2.50 mm"
equation "d31 = -adsk_phildepth"
equation "adsk_phildepth = 1.30 mm"
equation "d66 = adsk_headdia"
equation "d68 = adsk_nomlen"
equation "d71 = adsk_headh"
equation "d72 = adsk_philwidth"
equation "d76 = -adsk_phildepth"
equation "d79 = adsk_headh"
equation "adsk_thrlen = 8.50 mm"
equation "d84 = adsk_thrlen"
equation "adsk_startlen = 0.306725 mm"
equation "adsk_endpointdia = 2.38655 mm"
equation "d94 = adsk_nomdia * 0.51"
equation "d95 = adsk_startlen"
equation "d96 = adsk_endpointdia / 2"
equation "adsk_headtoprad = 0.10 mm"
equation "d102 = adsk_headtoprad"
equation "adsk_midfillet = 0.30 mm"
equation "d107 = adsk_midfillet"
